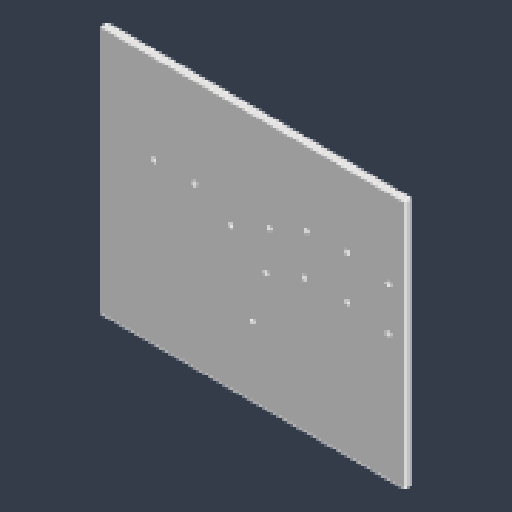
# Autodesk Inventor part: Top Plate
Saved by Autodesk Inventor 2023.4 (Build 274418000, 418)
## iProperties
Created: 2024-02-20
Part Number: Top Plate
Material: Generic
Document SubType Name: Modeling
Designer: JoaoSilva
Density: 1 g/cm^3
Appearance: Default
Author: JoaoSilva
Autodesk Inventor part; units mm, degrees
ref_plane "YZ Plane" through (0, 0, 0) normal (1, 0, 0) x (0, 1, 0)
ref_plane "XZ Plane" through (0, 0, 0) normal (0, 1, 0) x (-1, 0, 0)
ref_plane "XY Plane" through (0, 0, 0) normal (0, 0, 1) x (1, 0, 0)
sketch "Sketch1" plane through (0, 0, 0) normal (0, 0, 1) x (1, 0, 0)
  line L0 (-110, 90) -> (110, 90)
  line L1 (110, 90) -> (110, -90)
  line L2 (110, -90) -> (-110, -90)
  line L3 (-110, -90) -> (-110, 90)
  line L4 (-110, 90) -> (110, -90) construction
  line L5 (110, 90) -> (-110, -90) construction
  point P0 (0, 0)
  dimension "d0" = 220
  dimension "d1" = 180
  constraints: 12 end point, 2 midpoint, 2 parallel, 1 horizontal, 1 perpendicular
  measures "d0" distance of L0.start L0.end
  measures "d1" distance of L2.end L0.start
extrude "Extrusion1" add sketch "Sketch1" along normal blind 5
sketch "Sketch2" plane through (0, 0, 5) normal (0, 0, 1) x (1, 0, 0)
  line L0 (-110, -90) -> (110, -90) projected
  point P0 (0, 0)
  point P1 (0, -39.6)
  point P2 (-15.5, 12.8)
  point P3 (-41.8, 25.7)
  point P4 (-71.3, 25.6)
  point P5 (9.7, -4.6)
  point P6 (12.3, 24.8)
  point P7 (37.5, 6.4)
  point P8 (39.2, 36.5)
  point P9 (68.8, 6.7)
  point P10 (68.8, 37.7)
  point P11 (98.3, 1.7)
  point P12 (98.3, 32.7)
  dimension "d4" = 50.4
  dimension "d5" = 15.5
  dimension "d6" = 26.3
  dimension "d7" = 29.5
  dimension "d11" = 52.4
  dimension "d12" = 65.3
  dimension "d13" = 65.2
  dimension "d14" = 9.7
  dimension "d15" = 29.4
  dimension "d16" = 2.6
  dimension "d17" = 26.9
  dimension "d18" = 29.6
  dimension "d19" = 29.5
  dimension "d20" = 1.7
  dimension "d22" = 46
  dimension "d23" = 30.1
  dimension "d24" = 96.7
  dimension "d25" = 91.7
  dimension "d26" = 31
  dimension "d27" = 31
  dimension "d28" = 35
  constraints: 3 vertical alignment
  measures "d4" distance from line of L0 point (0, -39.6)
  measures "d5" horizontal distance of point (0, -39.6) point (-15.5, 12.8)
  measures "d6" horizontal distance of point (-41.8, 25.7) point (-15.5, 12.8)
  measures "d7" horizontal distance of point (-71.3, 25.6) point (-41.8, 25.7)
  measures "d11" vertical distance of point (0, -39.6) point (-15.5, 12.8)
  measures "d12" vertical distance of point (0, -39.6) point (-41.8, 25.7)
  measures "d13" vertical distance of point (-71.3, 25.6) point (0, -39.6)
  measures "d14" horizontal distance of point (9.7, -4.6) point (0, -39.6)
  measures "d15" vertical distance of point (12.3, 24.8) point (9.7, -4.6)
  measures "d16" horizontal distance of point (12.3, 24.8) point (9.7, -4.6)
  measures "d17" horizontal distance of point (39.2, 36.5) point (12.3, 24.8)
  measures "d18" horizontal distance of point (68.8, 37.7) point (39.2, 36.5)
  measures "d19" horizontal distance of point (98.3, 32.7) point (68.8, 37.7)
  measures "d20" horizontal distance of point (39.2, 36.5) point (37.5, 6.4)
  measures "d22" vertical distance of point (37.5, 6.4) point (0, -39.6)
  measures "d23" vertical distance of point (39.2, 36.5) point (37.5, 6.4)
  measures "d24" distance from line of L0 point (68.8, 6.7)
  measures "d25" distance from line of L0 point (98.3, 1.7)
  measures "d26" distance of point (98.3, 32.7) point (98.3, 1.7)
  measures "d27" distance of point (68.8, 6.7) point (68.8, 37.7)
  measures "d28" vertical distance of point (9.7, -4.6) point (0, -39.6)
hole "Hole1" at (0, -39.6, 5) at (-15.5, 12.8, 5) at (-41.8, 25.7, 5) at (-71.3, 25.6, 5) at (9.7, -4.6, 5) at (12.3, 24.8, 5) at (37.5, 6.4, 5) at (39.2, 36.5, 5) at (68.8, 6.7, 5) at (68.8, 37.7, 5) at (98.3, 1.7, 5) at (98.3, 32.7, 5) direction (0, 0, -1) diameter 3 end through all
sketch "Sketch3" plane through (0, 0, 5) normal (0, 0, 1) x (1, 0, 0)
  circle A0 centre (98.3, 1.7) radius 1.5 construction
  circle A1 centre (68.8, 6.7) radius 1.5 construction
  circle A2 centre (37.5, 6.4) radius 1.5 construction
  circle A3 centre (9.7, -4.6) radius 1.5 construction
  circle A4 centre (-41.8, 25.7) radius 1.5 construction
  circle A5 centre (0, -39.6) radius 1.5 construction
  circle A6 centre (-15.5, 12.8) radius 1.5 construction
  circle A7 centre (-71.3, 25.6) radius 1.5 construction
  circle A8 centre (12.3, 24.8) radius 1.5 construction
  circle A9 centre (39.2, 36.5) radius 1.5 construction
  circle A10 centre (68.8, 37.7) radius 1.5 construction
  circle A11 centre (98.3, 32.7) radius 1.5 construction
  line L0 (-110, -90) -> (110, -90) projected
  line L1 (110, -90) -> (110, 90) projected
  line L2 (110, 90) -> (-110, 90) projected
  line L3 (-110, 90) -> (-110, -90) projected
  line L4 (7, -32.6) -> (-7, -32.6)
  line L5 (-7, -32.6) -> (-7, -46.6)
  line L6 (-7, -46.6) -> (7, -46.6)
  line L7 (7, -46.6) -> (7, -32.6)
  circle A12 centre (0, -39.6) radius 1.5 construction
  line L8 (7, -32.6) -> (-7, -46.6) construction
  line L9 (-7, -32.6) -> (7, -46.6) construction
  line L10 (-8.5, 19.8) -> (-22.5, 19.8)
  line L11 (-22.5, 19.8) -> (-22.5, 5.8)
  line L12 (-22.5, 5.8) -> (-8.5, 5.8)
  line L13 (-8.5, 5.8) -> (-8.5, 19.8)
  line L14 (-8.5, 19.8) -> (-22.5, 5.8) construction
  line L15 (-22.5, 19.8) -> (-8.5, 5.8) construction
  line L16 (-34.8, 32.7) -> (-48.8, 32.7)
  line L17 (-48.8, 32.7) -> (-48.8, 18.7)
  line L18 (-48.8, 18.7) -> (-34.8, 18.7)
  line L19 (-34.8, 18.7) -> (-34.8, 32.7)
  line L20 (-34.8, 32.7) -> (-48.8, 18.7) construction
  line L21 (-48.8, 32.7) -> (-34.8, 18.7) construction
  line L22 (-64.3, 32.6) -> (-78.3, 32.6)
  line L23 (-78.3, 32.6) -> (-78.3, 18.6)
  line L24 (-78.3, 18.6) -> (-64.3, 18.6)
  line L25 (-64.3, 18.6) -> (-64.3, 32.6)
  line L26 (-64.3, 32.6) -> (-78.3, 18.6) construction
  line L27 (-78.3, 32.6) -> (-64.3, 18.6) construction
  line L28 (2.7, 2.4) -> (2.7, -11.6)
  line L29 (16.7, 2.4) -> (2.7, 2.4)
  line L30 (2.7, 2.4) -> (16.7, -11.6) construction
  line L31 (2.7, -11.6) -> (16.7, -11.6)
  line L32 (16.7, 2.4) -> (2.7, -11.6) construction
  line L33 (16.7, -11.6) -> (16.7, 2.4)
  line L34 (5.3, 31.8) -> (5.3, 17.8)
  line L35 (19.3, 31.8) -> (5.3, 31.8)
  line L36 (5.3, 31.8) -> (19.3, 17.8) construction
  line L37 (5.3, 17.8) -> (19.3, 17.8)
  line L38 (19.3, 31.8) -> (5.3, 17.8) construction
  line L39 (19.3, 17.8) -> (19.3, 31.8)
  line L40 (30.5, 13.4) -> (30.5, -0.6)
  line L41 (44.5, 13.4) -> (30.5, 13.4)
  line L42 (30.5, 13.4) -> (44.5, -0.6) construction
  line L43 (30.5, -0.6) -> (44.5, -0.6)
  line L44 (44.5, 13.4) -> (30.5, -0.6) construction
  line L45 (44.5, -0.6) -> (44.5, 13.4)
  line L46 (32.2, 43.5) -> (32.2, 29.5)
  line L47 (46.2, 43.5) -> (32.2, 43.5)
  line L48 (32.2, 43.5) -> (46.2, 29.5) construction
  line L49 (32.2, 29.5) -> (46.2, 29.5)
  line L50 (46.2, 43.5) -> (32.2, 29.5) construction
  line L51 (46.2, 29.5) -> (46.2, 43.5)
  line L52 (61.8, 13.7) -> (61.8, -0.3)
  line L53 (75.8, 13.7) -> (61.8, 13.7)
  line L54 (61.8, 13.7) -> (75.8, -0.3) construction
  line L55 (61.8, -0.3) -> (75.8, -0.3)
  line L56 (75.8, 13.7) -> (61.8, -0.3) construction
  line L57 (75.8, -0.3) -> (75.8, 13.7)
  line L58 (61.8, 44.7) -> (61.8, 30.7)
  line L59 (75.8, 44.7) -> (61.8, 44.7)
  line L60 (61.8, 44.7) -> (75.8, 30.7) construction
  line L61 (61.8, 30.7) -> (75.8, 30.7)
  line L62 (75.8, 44.7) -> (61.8, 30.7) construction
  line L63 (75.8, 30.7) -> (75.8, 44.7)
  line L64 (91.3, 8.7) -> (91.3, -5.3)
  line L65 (105.3, 8.7) -> (91.3, 8.7)
  line L66 (91.3, 8.7) -> (105.3, -5.3) construction
  line L67 (91.3, -5.3) -> (105.3, -5.3)
  line L68 (105.3, 8.7) -> (91.3, -5.3) construction
  line L69 (105.3, -5.3) -> (105.3, 8.7)
  line L70 (91.3, 39.7) -> (91.3, 25.7)
  line L71 (105.3, 39.7) -> (91.3, 39.7)
  line L72 (91.3, 39.7) -> (105.3, 25.7) construction
  line L73 (91.3, 25.7) -> (105.3, 25.7)
  line L74 (105.3, 39.7) -> (91.3, 25.7) construction
  line L75 (105.3, 25.7) -> (105.3, 39.7)
  point P0 (0, 0)
  point P1 (-15.5, 12.8)
  point P2 (9.7, -4.6)
  point P3 (37.5, 6.4)
  point P4 (68.8, 6.7)
  point P5 (68.8, 37.7)
  point P6 (98.3, 1.7)
  dimension "d36" = 14
  constraints: 144 end point, 24 midpoint, 24 parallel, 23 equal length, 12 horizontal, 12 perpendicular, 11 coincident
  measures "d36" distance of L6.end L5.end
extrude "Extrusion2" cut sketch "Sketch3" against normal through all contours L7 L6 L5 L4 | L13 L12 L11 L10 | L19 L18 L17 L16 | L25 L24 L23 L22 | L29 L33 L31 L28 | L35 L39 L37 L34 | L41 L45 L43 L40 | L47 L51 L49 L46 | L53 L57 L55 L52 | L59 L63 L61 L58 | L65 L69 L67 L64 | L71 L75 L73 L70
sketch "Sketch4" plane through (0, 0, 0) normal (0, 0, -1) x (-1, 0, 0)
  line L0 (8.5, 5.8) -> (8.5, 19.8) construction
  line L1 (8.5, 19.8) -> (22.5, 19.8) construction
  line L2 (22.5, 19.8) -> (22.5, 5.8) construction
  line L3 (22.5, 5.8) -> (8.5, 5.8) construction
  line L4 (-46.2, 29.5) -> (-46.2, 43.5) construction
  line L5 (-46.2, 43.5) -> (-32.2, 43.5) construction
  line L6 (-32.2, 43.5) -> (-32.2, 29.5) construction
  line L7 (-32.2, 29.5) -> (-46.2, 29.5) construction
  line L8 (-105.3, 25.7) -> (-105.3, 39.7) construction
  line L9 (-105.3, 39.7) -> (-91.3, 39.7) construction
  line L10 (-91.3, 39.7) -> (-91.3, 25.7) construction
  line L11 (-91.3, 25.7) -> (-105.3, 25.7) construction
  line L12 (-75.8, 30.7) -> (-75.8, 44.7) construction
  line L13 (-75.8, 44.7) -> (-61.8, 44.7) construction
  line L14 (-61.8, 44.7) -> (-61.8, 30.7) construction
  line L15 (-61.8, 30.7) -> (-75.8, 30.7) construction
  line L16 (-19.3, 17.8) -> (-19.3, 31.8) construction
  line L17 (-19.3, 31.8) -> (-5.3, 31.8) construction
  line L18 (-5.3, 31.8) -> (-5.3, 17.8) construction
  line L19 (-5.3, 17.8) -> (-19.3, 17.8) construction
  line L20 (34.8, 18.7) -> (34.8, 32.7) construction
  line L21 (34.8, 32.7) -> (48.8, 32.7) construction
  line L22 (48.8, 32.7) -> (48.8, 18.7) construction
  line L23 (48.8, 18.7) -> (34.8, 18.7) construction
  line L24 (-16.7, -11.6) -> (-16.7, 2.4) construction
  line L25 (-16.7, 2.4) -> (-2.7, 2.4) construction
  line L26 (-2.7, 2.4) -> (-2.7, -11.6) construction
  line L27 (-2.7, -11.6) -> (-16.7, -11.6) construction
  line L28 (-44.5, -0.6) -> (-44.5, 13.4) construction
  line L29 (-44.5, 13.4) -> (-30.5, 13.4) construction
  line L30 (-30.5, 13.4) -> (-30.5, -0.6) construction
  line L31 (-30.5, -0.6) -> (-44.5, -0.6) construction
  line L32 (-105.3, -5.3) -> (-105.3, 8.7) construction
  line L33 (-105.3, 8.7) -> (-91.3, 8.7) construction
  line L34 (-91.3, 8.7) -> (-91.3, -5.3) construction
  line L35 (-91.3, -5.3) -> (-105.3, -5.3) construction
  line L36 (-75.8, -0.3) -> (-75.8, 13.7) construction
  line L37 (-75.8, 13.7) -> (-61.8, 13.7) construction
  line L38 (-61.8, 13.7) -> (-61.8, -0.3) construction
  line L39 (-61.8, -0.3) -> (-75.8, -0.3) construction
  line L40 (7, -46.6) -> (-7, -46.6) construction
  line L41 (-7, -46.6) -> (-7, -32.6) construction
  line L42 (-7, -32.6) -> (7, -32.6) construction
  line L43 (7, -32.6) -> (7, -46.6) construction
  line L44 (64.3, 18.6) -> (64.3, 32.6) construction
  line L45 (64.3, 32.6) -> (78.3, 32.6) construction
  line L46 (78.3, 32.6) -> (78.3, 18.6) construction
  line L47 (78.3, 18.6) -> (64.3, 18.6) construction
  line L48 (110, -90) -> (-110, -90) construction
  line L49 (110, 90) -> (110, -90) construction
  line L50 (-110, 90) -> (110, 90) construction
  line L51 (-110, -90) -> (-110, 90) construction
  line L52 (-7.6, -47.2) -> (7.6, -47.2)
  line L53 (7.6, -47.2) -> (7.6, -32)
  line L54 (7.6, -32) -> (-7.6, -32)
  line L55 (-7.6, -32) -> (-7.6, -47.2)
  line L56 (-7.6, -47.2) -> (7.6, -32) construction
  line L57 (7.6, -47.2) -> (-7.6, -32) construction
  line L58 (7.9, 5.2) -> (23.1, 5.2)
  line L59 (23.1, 5.2) -> (23.1, 20.4)
  line L60 (23.1, 20.4) -> (7.9, 20.4)
  line L61 (7.9, 20.4) -> (7.9, 5.2)
  line L62 (7.9, 5.2) -> (23.1, 20.4) construction
  line L63 (23.1, 5.2) -> (7.9, 20.4) construction
  line L64 (34.2, 18.1) -> (49.4, 18.1)
  line L65 (49.4, 18.1) -> (49.4, 33.3)
  line L66 (49.4, 33.3) -> (34.2, 33.3)
  line L67 (34.2, 33.3) -> (34.2, 18.1)
  line L68 (34.2, 18.1) -> (49.4, 33.3) construction
  line L69 (49.4, 18.1) -> (34.2, 33.3) construction
  line L70 (63.7, 18) -> (78.9, 18)
  line L71 (78.9, 18) -> (78.9, 33.2)
  line L72 (78.9, 33.2) -> (63.7, 33.2)
  line L73 (63.7, 33.2) -> (63.7, 18)
  line L74 (63.7, 18) -> (78.9, 33.2) construction
  line L75 (78.9, 18) -> (63.7, 33.2) construction
  line L76 (-2.1, -12.2) -> (-17.3, 3) construction
  line L77 (-2.1, -12.2) -> (-2.1, 3)
  line L78 (-17.3, -12.2) -> (-2.1, 3) construction
  line L79 (-17.3, -12.2) -> (-2.1, -12.2)
  line L80 (-17.3, 3) -> (-17.3, -12.2)
  line L81 (-2.1, 3) -> (-17.3, 3)
  line L82 (-4.7, 17.2) -> (-19.9, 32.4) construction
  line L83 (-4.7, 17.2) -> (-4.7, 32.4)
  line L84 (-19.9, 17.2) -> (-4.7, 32.4) construction
  line L85 (-19.9, 17.2) -> (-4.7, 17.2)
  line L86 (-19.9, 32.4) -> (-19.9, 17.2)
  line L87 (-4.7, 32.4) -> (-19.9, 32.4)
  line L88 (-29.9, -1.2) -> (-45.1, 14) construction
  line L89 (-29.9, -1.2) -> (-29.9, 14)
  line L90 (-45.1, -1.2) -> (-29.9, 14) construction
  line L91 (-45.1, -1.2) -> (-29.9, -1.2)
  line L92 (-45.1, 14) -> (-45.1, -1.2)
  line L93 (-29.9, 14) -> (-45.1, 14)
  line L94 (-31.6, 28.9) -> (-46.8, 44.1) construction
  line L95 (-31.6, 28.9) -> (-31.6, 44.1)
  line L96 (-46.8, 28.9) -> (-31.6, 44.1) construction
  line L97 (-46.8, 28.9) -> (-31.6, 28.9)
  line L98 (-46.8, 44.1) -> (-46.8, 28.9)
  line L99 (-31.6, 44.1) -> (-46.8, 44.1)
  line L100 (-61.2, -0.9) -> (-76.4, 14.3) construction
  line L101 (-61.2, -0.9) -> (-61.2, 14.3)
  line L102 (-76.4, -0.9) -> (-61.2, 14.3) construction
  line L103 (-76.4, -0.9) -> (-61.2, -0.9)
  line L104 (-76.4, 14.3) -> (-76.4, -0.9)
  line L105 (-61.2, 14.3) -> (-76.4, 14.3)
  line L106 (-61.2, 30.1) -> (-76.4, 45.3) construction
  line L107 (-61.2, 30.1) -> (-61.2, 45.3)
  line L108 (-76.4, 30.1) -> (-61.2, 45.3) construction
  line L109 (-76.4, 30.1) -> (-61.2, 30.1)
  line L110 (-76.4, 45.3) -> (-76.4, 30.1)
  line L111 (-61.2, 45.3) -> (-76.4, 45.3)
  line L112 (-90.7, 25.1) -> (-105.9, 40.3) construction
  line L113 (-90.7, 25.1) -> (-90.7, 40.3)
  line L114 (-105.9, 25.1) -> (-90.7, 40.3) construction
  line L115 (-105.9, 25.1) -> (-90.7, 25.1)
  line L116 (-105.9, 40.3) -> (-105.9, 25.1)
  line L117 (-90.7, 40.3) -> (-105.9, 40.3)
  line L118 (-90.7, -5.9) -> (-105.9, 9.3) construction
  line L119 (-90.7, -5.9) -> (-90.7, 9.3)
  line L120 (-105.9, -5.9) -> (-90.7, 9.3) construction
  line L121 (-105.9, -5.9) -> (-90.7, -5.9)
  line L122 (-105.9, 9.3) -> (-105.9, -5.9)
  line L123 (-90.7, 9.3) -> (-105.9, 9.3)
  point P0 (0, 0)
  point P1 (0, -39.6)
  point P2 (15.5, 12.8)
  point P3 (41.8, 25.7)
  point P4 (71.3, 25.6)
  point P5 (-9.7, -4.6)
  point P6 (-12.3, 24.8)
  point P7 (-37.5, 6.4)
  point P8 (-39.2, 36.5)
  point P9 (-68.8, 6.7)
  point P10 (-68.8, 37.7)
  point P11 (-98.3, 32.7)
  point P12 (-98.3, 1.7)
  point P13 (0, -32.6)
  point P14 (15.5, 19.8)
  point P15 (41.8, 32.7)
  point P16 (71.3, 32.6)
  point P17 (-9.7, 2.4)
  point P18 (-12.3, 31.8)
  point P19 (-39.2, 43.5)
  point P20 (-68.8, 44.7)
  point P21 (-37.5, 13.4)
  point P22 (-68.8, 13.7)
  point P23 (-98.3, 8.7)
  point P24 (-98.3, 39.7)
  point P25 (-91.3, 32.7)
  point P26 (-91.3, 1.7)
  point P27 (-61.8, 6.7)
  point P28 (-61.8, 37.7)
  point P29 (-46.2, 36.5)
  point P30 (-30.5, 6.4)
  point P31 (-5.3, 24.8)
  point P32 (-2.7, -4.6)
  point P33 (22.5, 12.8)
  point P34 (48.8, 25.7)
  point P35 (78.3, 25.6)
  point P36 (7, -39.6)
  dimension "d46" = 15.2
  constraints: 144 end point, 48 midpoint, 24 parallel, 23 equal length, 12 horizontal, 12 horizontal alignment, 12 perpendicular, 12 vertical alignment
  measures "d46" distance of L54.end L53.end
extrude "Extrusion3" cut sketch "Sketch4" against normal blind 3.6
body "Solid1"
